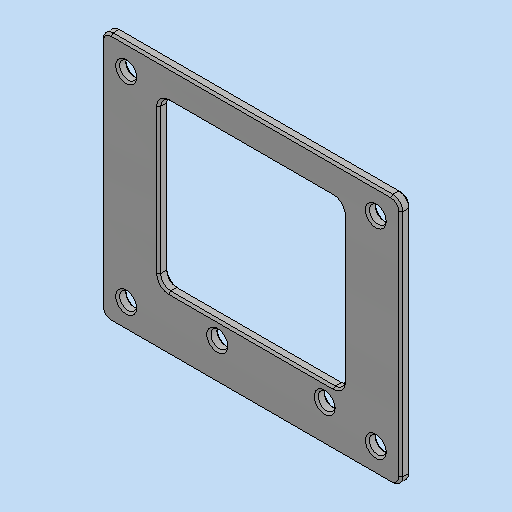
# Autodesk Inventor part: bradboardclip
Saved by Autodesk Inventor 2025 (Build 290162000, 162)
## iProperties
Created: 2024-12-25
Part Number: bradboardclip
Material: ABS Plastic
Document SubType Name: Modeling
Designer: kuzmin
Density: 1.06 g/cm^3
Appearance: Light Gray
Author: kuzmin
Autodesk Inventor part; units mm, degrees
ref_plane "YZ Plane" through (0, 0, 0) normal (1, 0, 0) x (0, 1, 0)
ref_plane "XZ Plane" through (0, 0, 0) normal (0, 1, 0) x (-1, 0, 0)
ref_plane "XY Plane" through (0, 0, 0) normal (0, 0, 1) x (1, 0, 0)
sketch "Sketch1" plane through (0, 0, 0) normal (0, 0, 1) x (1, 0, 0)
  line L0 (-30, 25) -> (30, 25)
  line L1 (30, 25) -> (30, -25)
  line L2 (30, -25) -> (-30, -25)
  line L3 (-30, -25) -> (-30, 25)
  point P0 (0, 0)
  point P1 (30, 0)
  point P2 (0, 25)
  dimension "d0" = 60
  dimension "d1" = 50
  constraints: 8 end point, 2 midpoint, 2 parallel, 1 horizontal, 1 horizontal alignment, 1 perpendicular, 1 vertical alignment
  measures "d0" distance of L0.start L0.end
  measures "d1" distance of L0.end L1.end
extrude "Extrusion1" add sketch "Sketch1" along normal blind 2
fillet "Fillet1" radius 2 4 edges at (30, 25, 1) (-30, 25, 1) (30, -25, 1) (-30, -25, 1)
sketch "Sketch2" plane through (0, 0, 2) normal (0, 0, 1) x (1, 0, 0)
  line L0 (-25, 20) -> (25, 20) construction
  line L1 (25, 20) -> (25, -20) construction
  line L2 (25, -20) -> (-25, -20) construction
  line L3 (-25, -20) -> (-25, 20) construction
  point P0 (0, 0)
  point P1 (25, 0)
  point P2 (0, 20)
  dimension "d5" = 50
  dimension "d6" = 40
  constraints: 8 end point, 4 coincident, 2 midpoint, 2 parallel, 1 horizontal, 1 horizontal alignment, 1 perpendicular, 1 vertical alignment
  measures "d5" distance of L0.start L0.end
  measures "d6" distance of L0.end L1.end
hole "Hole1" at (-25, 20, 2) at (25, 20, 2) at (-25, -20, 2) at (25, -20, 2) direction (0, 0, -1) diameter 3.4 end through all
sketch "Sketch3" plane through (0, 0, 2) normal (0, 0, 1) x (1, 0, 0)
  line L0 (-18.5, 19) -> (18.5, 19)
  line L1 (18.5, 19) -> (18.5, -14)
  line L2 (18.5, -14) -> (-18.5, -14)
  line L3 (-18.5, -14) -> (-18.5, 19)
  point P0 (0, 0)
  point P1 (0, 19)
  dimension "d15" = 33
  dimension "d16" = 37
  dimension "d17" = 14
  constraints: 8 end point, 2 parallel, 1 horizontal, 1 midpoint, 1 perpendicular, 1 vertical alignment
  measures "d15" distance of L0.end L1.end
  measures "d16" distance of L0.start L0.end
  measures "d17" distance from line of point (0, 0) L2
extrude "Extrusion2" cut sketch "Sketch3" against normal blind 2
fillet "Fillet2" radius 2 4 edges at (-18.5, 19, 1) (18.5, 19, 1) (18.5, -14, 1) (-18.5, -14, 1)
sketch "Sketch4" plane through (0, 0, 2) normal (0, 0, 1) x (1, 0, 0)
  line L0 (-6.75, -17.5) -> (14.75, -17.5) construction
  line L1 (16.5, -14) -> (-16.5, -14) projected
  point P0 (0, 0)
  point P1 (4, -17.5)
  dimension "d21" = 21.5
  dimension "d22" = 3.5
  dimension "d33" = 4
  constraints: 2 coincident, 2 end point, 1 horizontal, 1 midpoint
  measures "d21" distance of L0.start L0.end
  measures "d22" distance between parallel lines of L1 L0
  measures "d33" horizontal distance of point (4, -17.5) point (0, 0)
hole "Hole2" at (-6.75, -17.5, 2) at (14.75, -17.5, 2) direction (0, 0, -1) diameter 3.4 end through all
chamfer "Chamfer1" distance 0.4 angle 45 44 edges at (0, 25, 2) (-29.4142, 24.4142, 2) (-30, 0, 2) (-29.4142, -24.4142, 2) (0, -25, 2) (29.4142, -24.4142, 2) (30, 0, 2) (29.4142, 24.4142, 2) (0, 25, 0) (-29.4142, 24.4142, 0) (-30, 0, 0) (-29.4142, -24.4142, 0) (0, -25, 0) (29.4142, -24.4142, 0) (30, 0, 0) (29.4142, 24.4142, 0) (-18.5, 2.5, 0) (-17.9142, -13.4142, 0) (0, -14, 0) (17.9142, -13.4142, 0) (18.5, 2.5, 0) (17.9142, 18.4142, 0) (0, 19, 0) (-17.9142, 18.4142, 0) (0, 19, 2) (17.9142, 18.4142, 2) (18.5, 2.5, 2) (17.9142, -13.4142, 2) (0, -14, 2) (-17.9142, -13.4142, 2) (-18.5, 2.5, 2) (-17.9142, 18.4142, 2) (-25, -18.3, 2) (25, -18.3, 2) (-25, 21.7, 2) (25, 21.7, 2) (-6.75, -15.8, 2) (14.75, -15.8, 2) (-25, -18.3, 0) (25, -18.3, 0) (-25, 21.7, 0) (25, 21.7, 0) (-6.75, -15.8, 0) (14.75, -15.8, 0)
body "Solid1"
